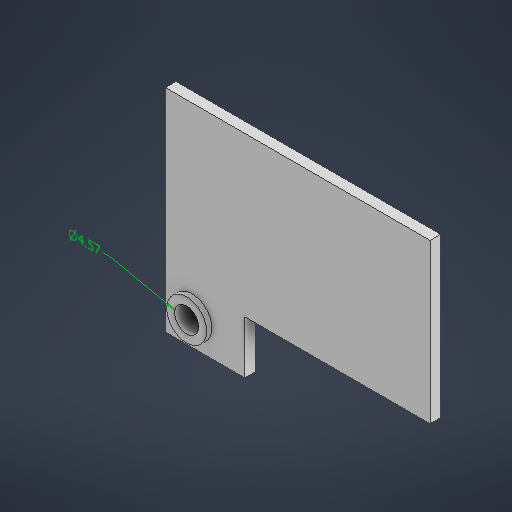
# Autodesk Inventor part: gate
Saved by Autodesk Inventor 2026.2 (Build 302298000, 298)
## iProperties
Created: 2026-02-24
Part Number: gate
Material: Generic
Document SubType Name: Modeling
Designer: danda
Density: 1 g/cm^3
Appearance: Default
Author: danda
Autodesk Inventor part; units mm, degrees
ref_plane "YZ Plane" through (0, 0, 0) normal (1, 0, 0) x (0, 1, 0)
ref_plane "XZ Plane" through (0, 0, 0) normal (0, 1, 0) x (-1, 0, 0)
ref_plane "XY Plane" through (0, 0, 0) normal (0, 0, 1) x (1, 0, 0)
sketch "Sketch1" plane through (0, 0, 0) normal (0, 0, 1) x (1, 0, 0)
  line L0 (0, 40) -> (50, 40)
  line L1 (50, 40) -> (50, 10)
  line L2 (7.5, 0) -> (0, 0)
  line L3 (0, 0) -> (0, 40)
  circle A0 centre (5, 5) radius 2.286
  circle A1 centre (5, 5) radius 3.786
  line L4 (50, 10) -> (15, 10)
  line L5 (15, 10) -> (15, 0)
  line L6 (15, 0) -> (0, 0)
  point P0 (0, 0)
  dimension "d2" = 0
  dimension "d3" = 0
  dimension "d4" = 4.572
  dimension "d7" = 1.5
  dimension "d13" = 30
  dimension "d14" = 50
  constraints: 14 end point, 2 centre point, 2 horizontal, 2 parallel, 2 perpendicular, 1 vertical
  measures "d2" distance of point (0, 0) L2.end
  measures "d3" distance from line of point (0, 0) L2
  measures "d4" diameter of A0
  measures "d7" radial gap between concentric circles of A0 A1
  measures "d13" distance of L0.end L1.end
  measures "d14" distance of L0.start L0.end
extrude "Extrusion1" add sketch "Sketch1" along normal mid plane 2 contours L0 L1 L4 L5 L6 L2 L3 | A1
extrude "Extrusion2" add sketch "Sketch1" along normal mid plane 4 contours A1
body "Solid1"
